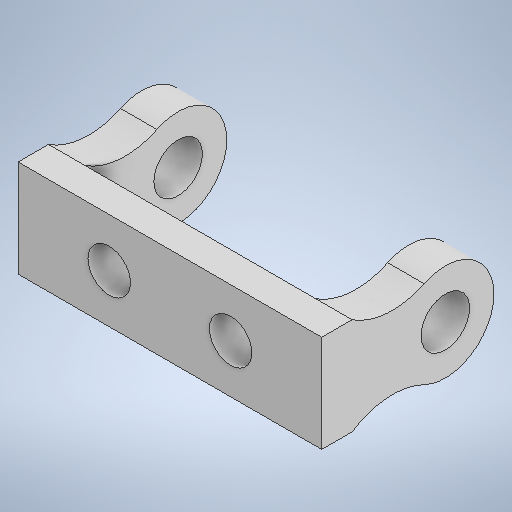
# Autodesk Inventor part: kipphebellagerbock
Saved by Autodesk Inventor 2025 (Build 290162010, 162A)
## iProperties
Created: 2024-04-30
Part Number: kipphebellagerbock
Material: Generisch
Document SubType Name: Modeling
Designer: ffogue
Density: 1 g/cm^3
Appearance: Vorgabe
Author: ffogue
Autodesk Inventor part; units mm, degrees
ref_plane "XZ Plane" through (0, 0, 0) normal (0, 1, 0) x (-1, 0, 0)
ref_plane "XY Plane" through (0, 0, 0) normal (0, 0, 1) x (1, 0, 0)
sketch "Skizze1" plane through (0, 0, 0) normal (1, 0, 0) x (0, 1, 0)
  line L0 (0, 0) -> (13, 0) construction
  line L1 (0, 0) -> (13, 0) construction
  line L2 (2.5, 4) -> (0, 4)
  line L3 (0, 4) -> (0, -4)
  line L4 (0, -4) -> (2.5, -4)
  line L5 (2.5, -4) -> (2.5, 4)
  arc A0 (2.5, 4) -> (8.432, 3.6) centre (5.8166, 9) ccw
  arc A1 (8.432, -3.6) -> (2.5, -4) centre (5.8166, -9) ccw
  arc A2 (8.432, -3.6) -> (8.432, 3.6) centre (10.1755, 0) ccw
  circle A3 centre (10.1755, 0) radius 2
  dimension "d7" = 13
  dimension "d9" = 2.5
  dimension "d10" = 12
  dimension "d11" = 12
  dimension "d15" = 8
  dimension "d16" = 18
  dimension "d21" = 4
  constraints: 12 end point, 6 point on circle, 4 centre point, 3 horizontal, 2 horizontal alignment, 2 parallel, 2 tangent, 1 coincident, 1 collinear, 1 midpoint, 1 perpendicular, 1 vertical alignment, 1 other
  measures "d7" distance of L0.start L0.end
  measures "d9" distance between parallel lines of L3 L5
  measures "d10" diameter of A0
  measures "d11" diameter of A1
  measures "d15" distance between parallel lines of L4 L2
  measures "d16" distance of A1.centre A0.centre
  measures "d21" diameter of A3
extrude "Extrusion1" add sketch "Skizze1" along normal blind 25 contours L5 L4 L3 L2
extrude "Extrusion2" add sketch "Skizze1" along normal blind 3 contours A0 A2 A1 L5
ref_plane "Arbeitsebene1" through (12.5, 0, 0) normal (1, 0, 0) x (0, 1, 0)
mirror "Spiegeln1" about plane through (12.5, 0, 0) normal (1, 0, 0) of "Extrusion2"
sketch "Skizze2" plane through (3, 2.5, 4) normal (0, 1, 0) x (1, 0, 0)
  line L0 (-3, 0) -> (-3, 8) projected
  line L1 (0, 0) -> (0, 8) projected
  point P0 (-3, 4)
  point P1 (4.5, 4)
  point P2 (14.5, 4)
  point P3 (-3, 4)
  point P4 (-3, 7.6)
  point P5 (-3, 0.4)
  point P6 (0, 7.6)
  point P7 (0, 0.4)
  dimension "d30" = 10
  dimension "d31" = 4.5
  constraints: 2 horizontal alignment, 1 midpoint
  measures "d30" distance of point (14.5, 4) point (4.5, 4)
  measures "d31" distance from line of point (4.5, 4) L1
hole "Bohrung1" at (7.5, 2.5, 0) at (17.5, 2.5, 0) direction (0, -1, 0) diameter 3.5 depth 2.5
